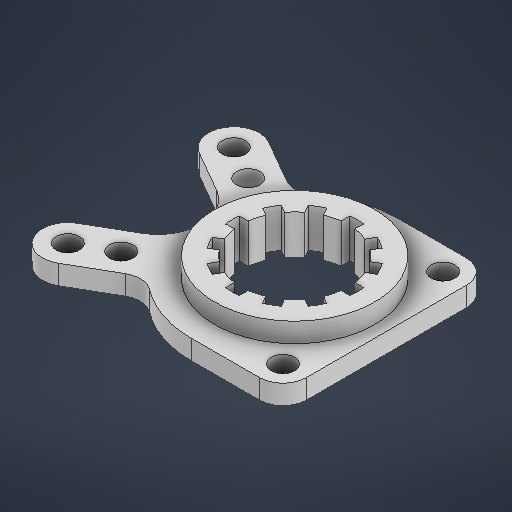
# Autodesk Inventor part: Splined_Flange_Mount
Saved by Autodesk Inventor 2026.1 (Build 301233020, 233B)
## iProperties
Created: 2026-02-15
Part Number: Splined_Flange_Mount
Material: Generic
Document SubType Name: Modeling
Designer: juanmiguelchungachun
Density: 1 g/cm^3
Appearance: Default
Author: juanmiguelchungachun
Autodesk Inventor part; units mm, degrees
ref_plane "YZ Plane" through (0, 0, 0) normal (1, 0, 0) x (0, 1, 0)
ref_plane "XZ Plane" through (0, 0, 0) normal (0, 1, 0) x (-1, 0, 0)
ref_plane "XY Plane" through (0, 0, 0) normal (0, 0, 1) x (1, 0, 0)
sketch "Sketch1" plane through (0, 0, 0) normal (0, 1, 0) x (-1, 0, 0)
  circle A0 centre (0, 0) radius 41
  line L0 (-47, 0) -> (-47, 41)
  line L1 (-35, 53) -> (0, 53)
  circle A1 centre (-35, 41) radius 6
  arc A2 (-35, 53) -> (-47, 41) centre (-35, 41) ccw
  circle A3 centre (73.6122, 42.5) radius 6
  circle A4 centre (56.2917, 32.5) radius 6
  line L2 (0, 0) -> (41, 0) construction
  line L3 (0, 0) -> (35.507, 20.5) construction
  line L4 (35.507, 20.5) -> (56.2917, 32.5) construction
  line L5 (56.2917, 32.5) -> (73.6122, 42.5) construction
  arc A5 (80.1122, 31.2417) -> (67.1122, 53.7583) centre (73.6122, 42.5) ccw
  line L6 (67.1122, 53.7583) -> (45.4615, 41.2583)
  line L7 (80.1122, 31.2417) -> (59, 19.0526)
  arc A6 (59, 19.0526) -> (48, 0) centre (70, 0) ccw
  arc A7 (32.1763, 42.1151) -> (45.4615, 41.2583) centre (39.4615, 51.6506) ccw
  line L8 (41, 0) -> (48, 0) construction
  circle A8 centre (73.6122, -42.5) radius 6
  circle A9 centre (56.2917, -32.5) radius 6
  arc A10 (67.1122, -53.7583) -> (80.1122, -31.2417) centre (73.6122, -42.5) ccw
  line L9 (67.1122, -53.7583) -> (45.4615, -41.2583)
  line L10 (80.1122, -31.2417) -> (59, -19.0526)
  arc A11 (48, 0) -> (59, -19.0526) centre (70, 0) ccw
  arc A12 (45.4615, -41.2583) -> (32.1763, -42.1151) centre (39.4615, -51.6506) ccw
  arc A13 (3.5, 31.808) -> (-3.5, 31.808) centre (0, 0) ccw
  arc A14 (10.6071, 25.372) -> (3.5, 27.2764) centre (0, 0) ccw
  line L11 (3.5, 31.808) -> (3.5, 27.2764)
  arc A15 (-12.8729, 29.2966) -> (-18.9351, 25.7966) centre (0, 0) ccw
  line L12 (-12.8729, 29.2966) -> (-10.6071, 25.372)
  arc A16 (-25.7966, 18.9351) -> (-29.2966, 12.8729) centre (0, 0) ccw
  line L13 (-25.7966, 18.9351) -> (-21.872, 16.6693)
  arc A17 (-31.808, 3.5) -> (-31.808, -3.5) centre (0, 0) ccw
  line L14 (-31.808, 3.5) -> (-27.2764, 3.5)
  arc A18 (-29.2966, -12.8729) -> (-25.7966, -18.9351) centre (0, 0) ccw
  line L15 (-29.2966, -12.8729) -> (-25.372, -10.6071)
  arc A19 (-18.9351, -25.7966) -> (-12.8729, -29.2966) centre (0, 0) ccw
  line L16 (-18.9351, -25.7966) -> (-16.6693, -21.872)
  arc A20 (-3.5, -31.808) -> (3.5, -31.808) centre (0, 0) ccw
  line L17 (-3.5, -31.808) -> (-3.5, -27.2764)
  arc A21 (12.8729, -29.2966) -> (18.9351, -25.7966) centre (0, 0) ccw
  line L18 (12.8729, -29.2966) -> (10.6071, -25.372)
  arc A22 (25.7966, -18.9351) -> (29.2966, -12.8729) centre (0, 0) ccw
  line L19 (25.7966, -18.9351) -> (21.872, -16.6693)
  arc A23 (31.808, -3.5) -> (31.808, 3.5) centre (0, 0) ccw
  line L20 (31.808, -3.5) -> (27.2764, -3.5)
  arc A24 (29.2966, 12.8729) -> (25.7966, 18.9351) centre (0, 0) ccw
  line L21 (29.2966, 12.8729) -> (25.372, 10.6071)
  arc A25 (18.9351, 25.7966) -> (12.8729, 29.2966) centre (0, 0) ccw
  line L22 (18.9351, 25.7966) -> (16.6693, 21.872)
  line L23 (10.6071, 25.372) -> (12.8729, 29.2966)
  arc A26 (-3.5, 27.2764) -> (-10.6071, 25.372) centre (0, 0) ccw
  line L24 (-3.5, 27.2764) -> (-3.5, 31.808)
  arc A27 (-16.6693, 21.872) -> (-21.872, 16.6693) centre (0, 0) ccw
  line L25 (-16.6693, 21.872) -> (-18.9351, 25.7966)
  arc A28 (-25.372, 10.6071) -> (-27.2764, 3.5) centre (0, 0) ccw
  line L26 (-25.372, 10.6071) -> (-29.2966, 12.8729)
  arc A29 (-27.2764, -3.5) -> (-25.372, -10.6071) centre (0, 0) ccw
  line L27 (-27.2764, -3.5) -> (-31.808, -3.5)
  arc A30 (-21.872, -16.6693) -> (-16.6693, -21.872) centre (0, 0) ccw
  line L28 (-21.872, -16.6693) -> (-25.7966, -18.9351)
  arc A31 (-10.6071, -25.372) -> (-3.5, -27.2764) centre (0, 0) ccw
  line L29 (-10.6071, -25.372) -> (-12.8729, -29.2966)
  arc A32 (3.5, -27.2764) -> (10.6071, -25.372) centre (0, 0) ccw
  line L30 (3.5, -27.2764) -> (3.5, -31.808)
  arc A33 (16.6693, -21.872) -> (21.872, -16.6693) centre (0, 0) ccw
  line L31 (16.6693, -21.872) -> (18.9351, -25.7966)
  arc A34 (25.372, -10.6071) -> (27.2764, -3.5) centre (0, 0) ccw
  line L32 (25.372, -10.6071) -> (29.2966, -12.8729)
  arc A35 (27.2764, 3.5) -> (25.372, 10.6071) centre (0, 0) ccw
  line L33 (27.2764, 3.5) -> (31.808, 3.5)
  arc A36 (21.872, 16.6693) -> (16.6693, 21.872) centre (0, 0) ccw
  line L34 (21.872, 16.6693) -> (25.7966, 18.9351)
  line L35 (-47, 0) -> (-47, -41)
  line L36 (-35, -53) -> (0, -53)
  circle A37 centre (-35, -41) radius 6
  arc A38 (-47, -41) -> (-35, -53) centre (-35, -41) ccw
  arc A39 (32.1763, 42.1151) -> (0, 53) centre (0, 0) ccw
  arc A40 (0, -53) -> (32.1763, -42.1151) centre (0, 0) ccw
  point P0 (25.7966, 18.9351)
  point P1 (31.808, 3.5)
  point P2 (29.2966, -12.8729)
  point P3 (18.9351, -25.7966)
  point P4 (3.5, -31.808)
  point P5 (-12.8729, -29.2966)
  point P6 (-25.7966, -18.9351)
  point P7 (-31.808, -3.5)
  point P8 (-29.2966, 12.8729)
  point P9 (-3.5, 31.808)
  dimension "d0" = 82
  dimension "d1" = 12
  dimension "d2" = 12
  dimension "d3" = 35
  dimension "d4" = 41
  dimension "d7" = 30
  dimension "d8" = 24
  dimension "d9" = 20
  dimension "d10" = 13
  dimension "d11" = 22
  dimension "d12" = 12
  dimension "d14" = 64
  dimension "d15" = 55
  dimension "d16" = 7
  dimension "d19" = 360
  dimension "d23" = 360
  dimension "d25" = 53
  constraints: 74 end point, 70 point on circle, 41 centre point, 14 symmetric about line, 8 coincident, 7 tangent, 3 horizontal alignment, 3 parallel, 2 collinear, 2 equal radius, 2 horizontal, 2 vertical, 1 perpendicular, 153 other
  measures "d0" diameter of A0
  measures "d1" diameter of A1
  measures "d2" radius of A2
  measures "d3" horizontal distance of A2.centre point (0, 0)
  measures "d4" vertical distance of point (0, 0) A1.centre
  measures "d7" angle of L2 L3
  measures "d8" distance of L3.end L4.end
  measures "d9" distance of L4.end L5.end
  measures "d10" radius of A5
  measures "d11" radius of A6
  measures "d12" radius of A7
  measures "d14" diameter of A13
  measures "d15" diameter of A14
  measures "d16" distance of L11.start A13.end
  measures "d25" radius of A40
extrude "Extrusion1" add sketch "Sketch1" along normal blind 10 contours L0 A2 L1 A39 A7 L6 A5 L7 A6 A11 L10 A10 L9 A12 A40 L36 A38 L35
extrude "Extrusion2" add sketch "Sketch1" along normal blind 20 contours A0
body "Solid1"
